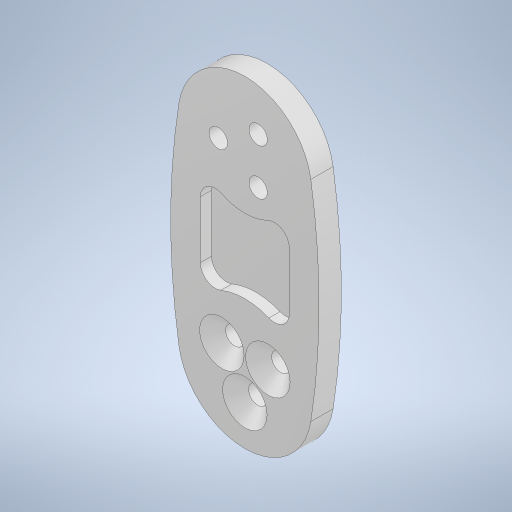
# Autodesk Inventor part: クランク_中間
Saved by Autodesk Inventor 2023.1 (Build 271208000, 208)
## iProperties
Created: 2022-01-08
Part Number: クランク_中間
Material: Aluminum 2014-T6
Document SubType Name: Modeling
Designer: acps
Density: 2.78927 g/cm^3
Appearance: Satin
Author: acps
Autodesk Inventor part; units mm, degrees
ref_plane "YZ Plane" through (0, 0, 0) normal (1, 0, 0) x (0, 1, 0)
ref_plane "XZ Plane" through (0, 0, 0) normal (0, 1, 0) x (-1, 0, 0)
ref_plane "XY Plane" through (0, 0, 0) normal (0, 0, 1) x (1, 0, 0)
sketch "Sketch2" plane through (0, 0, 0) normal (0, 0, 1) x (1, 0, 0)
  line L0 (-3.5796, 0) -> (-32.4095, 0) construction
  line L1 (-3.5796, 0) -> (-16.3075, 12.7279) construction
  line L2 (-3.5796, 0) -> (-16.3075, -12.7279) construction
  line L3 (-16.3075, 12.7279) -> (-16.3075, -12.7279) construction
  circle A0 centre (-14.5177, 15.8279) radius 1.25
  circle A1 centre (-14.5177, 15.8279) radius 3.1 construction
  circle A2 centre (-19.8871, 12.7279) radius 3.1 construction
  circle A3 centre (-19.8871, 12.7279) radius 1.25
  circle A4 centre (-14.5177, 9.6279) radius 3.1 construction
  circle A5 centre (-14.5177, 9.6279) radius 1.25
  circle A6 centre (-19.4075, -10.9381) radius 1.25
  circle A7 centre (-16.3075, -16.3075) radius 1.25
  circle A8 centre (-13.2075, -10.9381) radius 1.25
  line L4 (-16.3075, 12.7279) -> (-16.3075, -12.7279) construction
  line L5 (-25.3075, 12.7279) -> (-25.3075, -12.7279) construction
  line L6 (-7.3075, -12.7279) -> (-7.3075, 12.7279) construction
  arc A9 (-7.4179, 14.1335) -> (-25.1971, 14.1335) centre (-16.3075, 12.7279) ccw
  arc A10 (-25.1971, -14.1335) -> (-7.4179, -14.1335) centre (-16.3075, -12.7279) ccw
  arc A11 (-7.4179, -14.1335) -> (-7.4179, 14.1335) centre (-96.8075, 0) ccw
  arc A12 (-25.1971, 14.1335) -> (-25.1971, -14.1335) centre (64.1925, 0) ccw
  point P0 (0, 0)
  point P1 (-16.3075, 0)
  point P2 (-16.3075, 0)
  point P3 (-6.3075, 0)
  dimension "d20" = 18
  dimension "d21" = 18
  dimension "d22" = 90
  dimension "d23" = 2.5
  dimension "d24" = 6.2
  dimension "d25" = 360
  dimension "d26" = 2.5
  dimension "d27" = 360
  dimension "d28" = 6.2
  dimension "d29" = 9
  dimension "d31" = 10
  constraints: 18 end point, 13 centre point, 9 point on circle, 7 tangent, 3 coincident, 3 symmetric about line, 2 equal length, 2 midpoint, 1 horizontal, 1 horizontal alignment, 1 vertical, 1 vertical alignment, 22 other
  measures "d20" distance of L0.start L1.end
  measures "d21" distance of L0.start L2.end
  measures "d22" angle of L2 L1
  measures "d23" diameter of A0
  measures "d24" diameter of A1
  measures "d26" diameter of A6
  measures "d28" distance of A8.centre A6.centre
  measures "d29" radius of A10
  measures "d31" distance of point (-6.307, 0) point (-16.307, 0)
extrude "Extrusion1" add sketch "Sketch2" along normal blind 3
chamfer "Chamfer1" distance 1.75 angle 45 3 edges at (-14.4575, -10.9381, 3) (-20.6575, -10.9381, 3) (-17.5575, -16.3075, 3)
sketch "Sketch3" plane through (0, 0, 3) normal (0, 0, 1) x (1, 0, 0)
  circle A0 centre (-14.5177, 9.6279) radius 1.25 projected
  circle A1 centre (-19.8871, 12.7279) radius 1.25 projected
  arc A2 (-7.4179, -14.1335) -> (-7.4179, 14.1335) centre (-96.8075, 0) ccw projected
  circle A3 centre (-19.4075, -10.9381) radius 3 projected
  circle A4 centre (-13.2075, -10.9381) radius 3 projected
  circle A5 centre (-19.8871, 12.7279) radius 1.25 projected
  circle A6 centre (-14.5177, 15.8279) radius 1.25 projected
  circle A7 centre (-19.4075, -10.9381) radius 3 projected
  circle A8 centre (-14.5177, 15.8279) radius 1.25 projected
  circle A9 centre (-14.5177, 9.6279) radius 1.25 projected
  circle A10 centre (-19.8871, 12.7279) radius 1.25 projected
  arc A11 (-25.1971, -14.1335) -> (-7.4179, -14.1335) centre (-16.3075, -12.7279) ccw projected
  arc A12 (-7.4179, -14.1335) -> (-7.4179, 14.1335) centre (-96.8075, 0) ccw projected
  arc A13 (-7.4179, 14.1335) -> (-25.1971, 14.1335) centre (-16.3075, 12.7279) ccw projected
  arc A14 (-25.1971, 14.1335) -> (-25.1971, -14.1335) centre (64.1925, 0) ccw projected
  circle A15 centre (-13.2075, -10.9381) radius 3 projected
  circle A16 centre (-16.3075, -16.3075) radius 3 projected
  circle A17 centre (-16.3075, 12.7279) radius 7
  circle A18 centre (-16.3075, -12.7279) radius 8.5
  line L0 (-22.3075, 9.1224) -> (-22.3075, -6.7071)
  line L1 (-10.3075, 9.1224) -> (-10.3075, -6.7071)
  line L2 (-26.3075, 6.5531) -> (-26.3075, -6.806) construction
  line L3 (-6.3075, 6.3529) -> (-6.3075, -7.0063) construction
  point P0 (0, 0)
  dimension "d49" = 17
  dimension "d50" = 14
  dimension "d51" = 4
  dimension "d52" = 4
  constraints: 8 end point, 4 point on circle, 3 vertical, 2 centre point, 2 coincident, 2 tangent, 1 parallel
  measures "d49" diameter of A18
  measures "d50" diameter of A17
  measures "d51" distance between parallel lines of L2 L0
  measures "d52" distance between parallel lines of L1 L3
extrude "Extrusion2" cut sketch "Sketch3" against normal blind 1.5 contours A17 L1 A18 L0
fillet "フィレット1" radius 2 4 edges at (-22.3075, 9.1224, 2.25) (-22.3075, -6.7071, 2.25) (-10.3075, 9.1224, 2.25) (-10.3075, -6.7071, 2.25)
body "Solid1"
